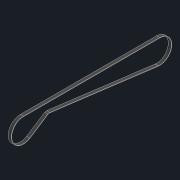
# Autodesk Inventor part: belt_1
Saved by Autodesk Inventor 2022 (Build 260153000, 153)
## iProperties
Created: 2021-07-18
Part Number: belt_1
Material: ゴム
Document SubType Name: Modeling
Designer: yuta0
Density: 0.93 g/cm^3
Appearance: ゴム - 黒
Mass: 8.55769 g
Surface Area: 248.449 cm^2
Volume: 9.20182 cm^3
購入先: ミスミ
在庫数: 0.0
Author: yuta0
Autodesk Inventor part; units mm, degrees
ref_plane "YZ Plane" through (0, 0, 0) normal (1, 0, 0) x (0, 1, 0)
ref_plane "XZ Plane" through (0, 0, 0) normal (0, 1, 0) x (-1, 0, 0)
ref_plane "XY Plane" through (0, 0, 0) normal (0, 0, 1) x (1, 0, 0)
sketch "スケッチ1" plane through (0, 0, 0) normal (1, 0, 0) x (0, 1, 0)
  arc A0 (38.1972, 0) -> (-32.0976, -20.7068) centre (0, 0) ccw
  arc A1 (-37.8876, -435.1467) -> (38.1972, -440) centre (0, -440) ccw
  arc A2 (6.9469, -85.1461) -> (5.5796, -79.1102) centre (-2, -84) ccw
  line L0 (5.5796, -79.1102) -> (-32.0976, -20.7068)
  line L1 (38.1972, -440) -> (38.1972, 0)
  line L2 (6.9469, -85.1461) -> (-37.8876, -435.1467)
  arc A3 (39.2172, 0) -> (-32.9547, -21.2597) centre (0, 0) ccw
  line L3 (-32.9547, -21.2597) -> (4.7225, -79.6632)
  arc A4 (5.9352, -85.0165) -> (4.7225, -79.6632) centre (-2, -84) ccw
  line L4 (5.9352, -85.0165) -> (-38.8993, -435.0171)
  arc A5 (-38.8993, -435.0171) -> (39.2172, -440) centre (0, -440) ccw
  line L5 (39.2172, -440) -> (39.2172, 0)
  arc A6 (37.7172, 0) -> (-31.6942, -20.4466) centre (0, 0) ccw
  line L6 (-31.6942, -20.4466) -> (5.983, -78.85)
  arc A7 (7.423, -85.2071) -> (5.983, -78.85) centre (-2, -84) ccw
  line L7 (7.423, -85.2071) -> (-37.4115, -435.2077)
  arc A8 (-37.4115, -435.2077) -> (37.7172, -440) centre (0, -440) ccw
  line L8 (37.7172, -440) -> (37.7172, 0)
  dimension "d0" = 76.3944
  dimension "d1" = 76.3944
  dimension "d2" = 440
  dimension "d25" = 8
  dimension "d26" = 84
  dimension "d30" = 2
  dimension "d31" = 1.5
  dimension "d32" = 0.48
  constraints: 18 end point, 18 point on circle, 9 centre point, 6 tangent, 1 coincident, 1 vertical alignment, 10 other
  measures "d0" diameter of A0
  measures "d1" diameter of A1
  measures "d2" distance of A0.centre A1.centre
  measures "d25" radius of A4
  measures "d26" vertical distance of point (0, 0) A2.centre
  measures "d30" horizontal distance of point (0, 0) A2.centre
  measures "d31" distance between parallel lines of L5 L8
  measures "d32" distance between parallel lines of L8 L1
extrude "押し出し1" add sketch "スケッチ1" along normal mid plane 10 contours L1 A1 L2 A2 L0 A0 | L5 A5 L4 A4 L3 A3
equation "\"d0\" = d1"
